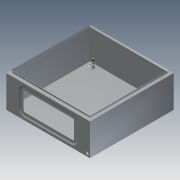
# Autodesk Inventor part: AE 1050_01_00
Saved by Autodesk Inventor 2016 (Build 200138000, 138)
## iProperties
Category: PARTsolutions
Company: RITTAL
Created: 2014-04-04
Part Number: AE 1050_01_00
Catalog Web Link: www.cadenas.de
Description: Gehäusekorpus AE-Gehäusekorpus AE
Vendor: RITTAL
Document SubType Name: Modeling
Designer: PARTuser1
Manufacturer: RITTAL
Density: 1 g/cm^3
Material: Generic
Appearance: RGB(195.00000357627781,201.00000321865156,196.00000351667384)
PSOL_IDENT_0: {$CADENAS_DATA\23d-libs\rittal\schaltschranksys\kompakt_schaltschr\ae\parts_ae\gehaeusekorpus_ae.prj
PSOL_IDENT_1: },187 {VTYP=3D},{NB=1050_01_00 (1)},{LINA=1050_01_00 (1)},{NN=Gehäusekorpus AE},{DATE=28.03.2014 09:
PSOL_IDENT_2: 17:10},{GEOMDATE=28.03.2014 09:16:00},{VERSION=},{LINEID=180},{LINESUBID=-1},{WBVAR=DETAIL}  {NB=105
PSOL_IDENT_3: 0_01_00 (1)},{LINA=1050_01_00 (1)},{KT=DUMMY},{BEST=1050},{VER=0},{SS=1.20},{DETAIL=1},{A=500.000},{
PSOL_IDENT_4: B=500.000},{C=210.000},{D=303.000},{E=113.000},{F=38.000},{G=30.000},{H=445.000},{I=355.000},{K=470.
PSOL_IDENT_5: 000},{P=410.000},{Q=449.000},{R=495.000},{S=495.000},{T=356.300},{U=425.000},{V=17.000},{W=438.000},
PSOL_IDENT_6: {X=411.000},{Y=423.000},{B1=500},{H1=500},{T1=210},{F1=449},{G1=470},{S1=2.5},{GEW=16.8},{VERS=1},{G
PSOL_IDENT_7: G=10.000},{AA=17.000},{BB=7.000},{CC=10.000},{RR=31.000}
CNS_NN: Gehäusekorpus AE
CNS_NT: Gehäusekorpus AE
CNS_NB: 1050_01_00 (1)
CNS_NBSYN: $BEST._01_00 ($DETAIL.)
CNS_LINA: 1050_01_00 (1)
CNS_BEST: 1050
CNS_VER: 0
CNS_SS: 1.20
CNS_DETAIL: 1
CNS_A: 500.000
CNS_B: 500.000
CNS_C: 210.000
CNS_D: 303.000
CNS_E: 113.000
CNS_F: 38.000
CNS_G: 30.000
CNS_H: 445.000
CNS_I: 355.000
CNS_K: 470.000
CNS_P: 410.000
CNS_Q: 449.000
CNS_R: 495.000
CNS_S: 495.000
CNS_T: 356.300
CNS_U: 425.000
CNS_V: 17.000
CNS_W: 438.000
CNS_X: 411.000
CNS_Y: 423.000
CNS_B1: 500
CNS_H1: 500
CNS_T1: 210
CNS_F1: 449
CNS_G1: 470
CNS_S1: 2.5
CNS_GEW: 16.8
CNS_VERS: 1
CNS_GG: 10.000
CNS_AA: 17.000
CNS_BB: 7.000
CNS_CC: 10.000
CNS_RR: 31.000
SUPPLIER: RITTAL
ARTICLENO: 1050_01_00 (1)
BOMINFO: 1050_01_00 (1)
CREATOR: CADENAS GmbH
Title: 1050_01_00 (1)
Author: Cadenas PARTsolutions
Comments: Gehäusekorpus AE
Autodesk Inventor part; units mm, degrees
sketch "Sketch_10" plane through (0, 0, 0) normal (0, 1, 0) x (-1, 0, 0)
  line L0 (250, -105) -> (250, 85)
  line L1 (250, 85) -> (-250, 85)
  line L2 (-250, 85) -> (-250, -105)
  line L3 (-250, -105) -> (250, -105)
  constraints: 8 end point
extrude "Extrusion1" add sketch "Sketch_10" along normal blind 500
sketch "Skizze_4" plane through (0, 0, 0) normal (1, 0, 0) x (0, 0, -1)
  line L0 (-210, 17) -> (0, 17)
  line L1 (0, 17) -> (0, 483)
  line L2 (0, 483) -> (-210, 483)
  line L3 (-210, 483) -> (-210, 17)
  constraints: 8 end point
extrude "Extrusion2" cut sketch "Skizze_4" along normal mid plane 465
sketch "Sketch_9" plane through (0, 0, 0) normal (1, 0, 0) x (0, 1, 0)
  line L0 (1.2, 83.8) -> (1.2, -103.8)
  line L1 (1.2, -103.8) -> (498.8, -103.8)
  line L2 (498.8, -103.8) -> (498.8, 83.8)
  line L3 (498.8, 83.8) -> (1.2, 83.8)
  constraints: 8 end point
extrude "Extrusion3" cut sketch "Sketch_9" along normal mid plane 497.6
sketch "Skizze_6" plane through (0, 0, 0) normal (1, 0, 0) x (0, 0, -1)
  line L0 (-103.9031, 11.333) -> (-103.9031, 10.1328)
  line L1 (-103.9031, 10.1328) -> (-83.8, 10.1328)
  line L2 (-83.8, 10.1328) -> (-83.8, 18)
  arc A0 (-83.8, 18) -> (-85.8, 20) centre (-85.8, 18) ccw
  line L3 (-85.8, 20) -> (-91.349, 20)
  arc A1 (-91.349, 20) -> (-92.5263, 19.6168) centre (-91.349, 18) ccw
  line L4 (-92.5263, 19.6168) -> (-103.9031, 11.333)
  constraints: 10 end point, 4 point on circle, 2 centre point
extrude "Extrusion4" add sketch "Skizze_6" along normal mid plane 478.4
sketch "Skizze_7" plane through (0, 0, 0) normal (1, 0, 0) x (0, 0, -1)
  line L0 (-103.9031, 488.667) -> (-92.5263, 480.3832)
  arc A0 (-92.5263, 480.3832) -> (-91.349, 480) centre (-91.349, 482) ccw
  line L1 (-91.349, 480) -> (-85.8, 480)
  arc A1 (-85.8, 480) -> (-83.8, 482) centre (-85.8, 482) ccw
  line L2 (-83.8, 482) -> (-83.8, 489.8672)
  line L3 (-83.8, 489.8672) -> (-103.9031, 489.8672)
  line L4 (-103.9031, 489.8672) -> (-103.9031, 488.667)
  constraints: 10 end point, 4 point on circle, 2 centre point
extrude "Extrusion5" add sketch "Skizze_7" along normal mid plane 476.4
sketch "Skizze_8" plane through (0, 250, 0) normal (0, 1, 0) x (1, 0, 0)
  line L0 (230, -85.8) -> (230, -91.349)
  arc A0 (230, -91.349) -> (230.3832, -92.5263) centre (232, -91.349) ccw
  line L1 (230.3832, -92.5263) -> (238.667, -103.9031)
  line L2 (238.667, -103.9031) -> (239.867, -103.9031)
  line L3 (239.867, -103.9031) -> (239.867, -83.8)
  line L4 (239.867, -83.8) -> (232, -83.8)
  arc A1 (232, -83.8) -> (230, -85.8) centre (232, -85.8) ccw
  constraints: 10 end point, 4 point on circle, 2 centre point
extrude "Extrusion6" add sketch "Skizze_8" along normal mid plane 481.4
sketch "Skizze_9" plane through (0, 250, 0) normal (0, 1, 0) x (1, 0, 0)
  line L0 (-240.6254, -103.9031) -> (-238.667, -103.9031)
  line L1 (-238.667, -103.9031) -> (-230.3832, -92.5263)
  arc A0 (-230.3832, -92.5263) -> (-230, -91.349) centre (-232, -91.349) ccw
  line L2 (-230, -91.349) -> (-230, -85.8)
  arc A1 (-230, -85.8) -> (-232, -83.8) centre (-232, -85.8) ccw
  line L3 (-232, -83.8) -> (-240.6254, -83.8)
  line L4 (-240.6254, -83.8) -> (-240.6254, -103.9031)
  constraints: 10 end point, 4 point on circle, 2 centre point
extrude "Extrusion7" add sketch "Skizze_9" along normal mid plane 481.4
sketch "Skizze_20" plane through (0, 0, 0) normal (1, 0, 0) x (0, 0, -1)
  line L0 (-296.7396, -2) -> (-85, -2)
  line L1 (-85, -2) -> (-85, 18)
  arc A0 (-85, 18) -> (-85.8, 18.8) centre (-85.8, 18) ccw
  line L2 (-85.8, 18.8) -> (-91.3601, 18.8)
  arc A1 (-91.3601, 18.8) -> (-91.8245, 18.6514) centre (-91.3601, 18) ccw
  line L3 (-91.8245, 18.6514) -> (-98.7083, 13.7444)
  line L4 (-98.7083, 13.7444) -> (-276.7396, 250)
  line L5 (-276.7396, 250) -> (-98.7083, 486.2556)
  line L6 (-98.7083, 486.2556) -> (-91.8245, 481.3486)
  arc A2 (-91.8245, 481.3486) -> (-91.3601, 481.2) centre (-91.3601, 482) ccw
  line L7 (-91.3601, 481.2) -> (-85.8, 481.2)
  arc A3 (-85.8, 481.2) -> (-85, 482) centre (-85.8, 482) ccw
  line L8 (-85, 482) -> (-85, 502)
  line L9 (-85, 502) -> (-296.7396, 502)
  line L10 (-296.7396, 502) -> (-296.7396, -2)
  constraints: 22 end point, 8 point on circle, 4 centre point
extrude "Extrusion8" cut sketch "Skizze_20" along normal mid plane 1476.4
sketch "Skizze_21" plane through (0, 250, 0) normal (0, 1, 0) x (1, 0, 0)
  line L0 (-251.2, -85) -> (-251.2, -296.7396)
  line L1 (-251.2, -296.7396) -> (251.2, -296.7396)
  line L2 (251.2, -296.7396) -> (251.2, -85)
  line L3 (251.2, -85) -> (232, -85)
  arc A0 (232, -85) -> (231.2, -85.8) centre (232, -85.8) ccw
  line L4 (231.2, -85.8) -> (231.2, -91.3601)
  arc A1 (231.2, -91.3601) -> (231.3486, -91.8245) centre (232, -91.3601) ccw
  line L5 (231.3486, -91.8245) -> (236.2556, -98.7083)
  line L6 (236.2556, -98.7083) -> (0, -276.7396)
  line L7 (0, -276.7396) -> (-236.2556, -98.7083)
  line L8 (-236.2556, -98.7083) -> (-231.3486, -91.8245)
  arc A2 (-231.3486, -91.8245) -> (-231.2, -91.3601) centre (-232, -91.3601) ccw
  line L9 (-231.2, -91.3601) -> (-231.2, -85.8)
  arc A3 (-231.2, -85.8) -> (-232, -85) centre (-232, -85.8) ccw
  line L10 (-232, -85) -> (-251.2, -85)
  constraints: 22 end point, 8 point on circle, 4 centre point
extrude "Extrusion9" cut sketch "Skizze_21" along normal mid plane 496.4
sketch "Sketch10" plane through (-250, 0, 85) normal (0, 0, 1) x (1, 0, 0)
  point P0 (490.3, 50.65)
hole "Drilling 1" at (240.3, 50.65, 85) direction (0, 0, -1) diameter 4.4 depth 1.2
sketch "Skizze_28" plane through (0, 0, 0) normal (0, 1, 0) x (1, 0, 0)
  line L0 (-182.9449, 50.4449) -> (-182.9449, -29.4449)
  arc A0 (-182.9449, -29.4449) -> (-134.9449, -77.4449) centre (-134.9449, -29.4449) ccw
  line L1 (-134.9449, -77.4449) -> (134.9449, -77.4449)
  arc A1 (134.9449, -77.4449) -> (182.9449, -29.4449) centre (134.9449, -29.4449) ccw
  line L2 (182.9449, -29.4449) -> (182.9449, 50.4449)
  arc A2 (182.9449, 50.4449) -> (134.9449, 98.4449) centre (134.9449, 50.4449) ccw
  line L3 (134.9449, 98.4449) -> (-134.9449, 98.4449)
  arc A3 (-134.9449, 98.4449) -> (-182.9449, 50.4449) centre (-134.9449, 50.4449) ccw
  constraints: 8 end point, 8 point on circle, 4 centre point
extrude "Extrusion10" cut sketch "Skizze_28" along normal blind 1.2
sketch "Skizze_29" plane through (0, 0, -10.5) normal (0, 0, 1) x (1, 0, 0)
  line L0 (147.5, 4) -> (167.6962, 4)
  arc A0 (168.5962, 3.7588) -> (167.6962, 4) centre (167.6962, 2.2) ccw
  line L1 (168.5962, 3.7588) -> (174.4105, 0.4019)
  arc A1 (174.4105, 0.4019) -> (175.9105, 0) centre (175.9105, 3) ccw
  line L2 (175.9105, 0) -> (182.9949, 0)
  line L3 (182.9949, 0) -> (182.9949, 1.2)
  line L4 (182.9949, 1.2) -> (175.9105, 1.2)
  arc A2 (175.0105, 1.4412) -> (175.9105, 1.2) centre (175.9105, 3) ccw
  line L5 (175.0105, 1.4412) -> (169.1962, 4.7981)
  arc A3 (169.1962, 4.7981) -> (167.6962, 5.2) centre (167.6962, 2.2) ccw
  line L6 (167.6962, 5.2) -> (147.5, 5.2)
  line L7 (147.5, 5.2) -> (147.5, 4)
  constraints: 16 end point, 8 point on circle, 4 centre point
extrude "Extrusion11" add sketch "Skizze_29" along normal mid plane 85
sketch "Skizze_30" plane through (0, 0, -10.5) normal (0, 0, 1) x (1, 0, 0)
  line L0 (-182.9949, 0) -> (-175.9105, 0)
  arc A0 (-175.9105, 0) -> (-174.4105, 0.4019) centre (-175.9105, 3) ccw
  line L1 (-174.4105, 0.4019) -> (-168.5962, 3.7588)
  arc A1 (-167.6962, 4) -> (-168.5962, 3.7588) centre (-167.6962, 2.2) ccw
  line L2 (-167.6962, 4) -> (-147.5, 4)
  line L3 (-147.5, 4) -> (-147.5, 5.2)
  line L4 (-147.5, 5.2) -> (-167.6962, 5.2)
  arc A2 (-167.6962, 5.2) -> (-169.1962, 4.7981) centre (-167.6962, 2.2) ccw
  line L5 (-169.1962, 4.7981) -> (-175.0105, 1.4412)
  arc A3 (-175.9105, 1.2) -> (-175.0105, 1.4412) centre (-175.9105, 3) ccw
  line L6 (-175.9105, 1.2) -> (-182.9949, 1.2)
  line L7 (-182.9949, 1.2) -> (-182.9949, 0)
  constraints: 16 end point, 8 point on circle, 4 centre point
extrude "Extrusion12" add sketch "Skizze_30" along normal mid plane 85
sketch "Skizze_31" plane through (0, 0, -53) normal (0, 0, 1) x (1, 0, 0)
  line L0 (137.5, -50) -> (137.5, 50)
  line L1 (147.5, 4) -> (167.6962, 4)
  arc A0 (168.5962, 3.7588) -> (167.6962, 4) centre (167.6962, 2.2) ccw
  line L2 (168.5962, 3.7588) -> (174.4105, 0.4019)
  arc A1 (174.4105, 0.4019) -> (175.9105, 0) centre (175.9105, 3) ccw
  line L3 (175.9105, 0) -> (182.9949, 0)
  line L4 (182.9949, 0) -> (182.9949, 1.2)
  line L5 (182.9949, 1.2) -> (175.9105, 1.2)
  arc A2 (175.0105, 1.4412) -> (175.9105, 1.2) centre (175.9105, 3) ccw
  line L6 (175.0105, 1.4412) -> (169.1962, 4.7981)
  arc A3 (169.1962, 4.7981) -> (167.6962, 5.2) centre (167.6962, 2.2) ccw
  line L7 (167.6962, 5.2) -> (147.5, 5.2)
  line L8 (147.5, 5.2) -> (147.5, 4)
  constraints: 18 end point, 8 point on circle, 4 centre point
revolve "Revolution1" add sketch "Skizze_31" angle 90 about axis through (137.5, -50, -53) along (0, 1, 0)
sketch "Skizze_32" plane through (0, 0, -53) normal (0, 0, 1) x (1, 0, 0)
  line L0 (-137.5, 4) -> (-137.5, -4)
  line L1 (-182.9949, 0) -> (-175.9105, 0)
  arc A0 (-175.9105, 0) -> (-174.4105, 0.4019) centre (-175.9105, 3) ccw
  line L2 (-174.4105, 0.4019) -> (-168.5962, 3.7588)
  arc A1 (-167.6962, 4) -> (-168.5962, 3.7588) centre (-167.6962, 2.2) ccw
  line L3 (-167.6962, 4) -> (-147.5, 4)
  line L4 (-147.5, 4) -> (-147.5, 5.2)
  line L5 (-147.5, 5.2) -> (-167.6962, 5.2)
  arc A2 (-167.6962, 5.2) -> (-169.1962, 4.7981) centre (-167.6962, 2.2) ccw
  line L6 (-169.1962, 4.7981) -> (-175.0105, 1.4412)
  arc A3 (-175.9105, 1.2) -> (-175.0105, 1.4412) centre (-175.9105, 3) ccw
  line L7 (-175.9105, 1.2) -> (-182.9949, 1.2)
  line L8 (-182.9949, 1.2) -> (-182.9949, 0)
  constraints: 18 end point, 8 point on circle, 4 centre point
revolve "Revolution2" add sketch "Skizze_32" angle 90 about axis through (-137.5, 4, -53) along (0, -1, 0)
sketch "Skizze_33" plane through (0, 0, 32) normal (0, 0, 1) x (1, 0, 0)
  line L0 (137.5, -50) -> (137.5, 50)
  line L1 (147.5, 4) -> (167.6962, 4)
  arc A0 (168.5962, 3.7588) -> (167.6962, 4) centre (167.6962, 2.2) ccw
  line L2 (168.5962, 3.7588) -> (174.4105, 0.4019)
  arc A1 (174.4105, 0.4019) -> (175.9105, 0) centre (175.9105, 3) ccw
  line L3 (175.9105, 0) -> (182.9949, 0)
  line L4 (182.9949, 0) -> (182.9949, 1.2)
  line L5 (182.9949, 1.2) -> (175.9105, 1.2)
  arc A2 (175.0105, 1.4412) -> (175.9105, 1.2) centre (175.9105, 3) ccw
  line L6 (175.0105, 1.4412) -> (169.1962, 4.7981)
  arc A3 (169.1962, 4.7981) -> (167.6962, 5.2) centre (167.6962, 2.2) ccw
  line L7 (167.6962, 5.2) -> (147.5, 5.2)
  line L8 (147.5, 5.2) -> (147.5, 4)
  constraints: 18 end point, 8 point on circle, 4 centre point
revolve "Revolution3" add sketch "Skizze_33" angle 90 about axis through (137.5, -50, 32) along (0, -1, 0)
sketch "Skizze_34" plane through (0, 0, 32) normal (0, 0, 1) x (1, 0, 0)
  line L0 (-137.5, 4) -> (-137.5, -4)
  line L1 (-182.9949, 0) -> (-175.9105, 0)
  arc A0 (-175.9105, 0) -> (-174.4105, 0.4019) centre (-175.9105, 3) ccw
  line L2 (-174.4105, 0.4019) -> (-168.5962, 3.7588)
  arc A1 (-167.6962, 4) -> (-168.5962, 3.7588) centre (-167.6962, 2.2) ccw
  line L3 (-167.6962, 4) -> (-147.5, 4)
  line L4 (-147.5, 4) -> (-147.5, 5.2)
  line L5 (-147.5, 5.2) -> (-167.6962, 5.2)
  arc A2 (-167.6962, 5.2) -> (-169.1962, 4.7981) centre (-167.6962, 2.2) ccw
  line L6 (-169.1962, 4.7981) -> (-175.0105, 1.4412)
  arc A3 (-175.9105, 1.2) -> (-175.0105, 1.4412) centre (-175.9105, 3) ccw
  line L7 (-175.9105, 1.2) -> (-182.9949, 1.2)
  line L8 (-182.9949, 1.2) -> (-182.9949, 0)
  constraints: 18 end point, 8 point on circle, 4 centre point
revolve "Revolution4" add sketch "Skizze_34" angle 90 about axis through (-137.5, 4, 32) along (0, 1, 0)
sketch "Skizze_35" plane through (0, 0, 0) normal (1, 0, 0) x (0, 0, -1)
  line L0 (63, 4) -> (83.1962, 4)
  arc A0 (84.0962, 3.7588) -> (83.1962, 4) centre (83.1962, 2.2) ccw
  line L1 (84.0962, 3.7588) -> (89.9105, 0.4019)
  arc A1 (89.9105, 0.4019) -> (91.4105, 0) centre (91.4105, 3) ccw
  line L2 (91.4105, 0) -> (98.4949, 0)
  line L3 (98.4949, 0) -> (98.4949, 1.2)
  line L4 (98.4949, 1.2) -> (91.4105, 1.2)
  arc A2 (90.5105, 1.4412) -> (91.4105, 1.2) centre (91.4105, 3) ccw
  line L5 (90.5105, 1.4412) -> (84.6962, 4.7981)
  arc A3 (84.6962, 4.7981) -> (83.1962, 5.2) centre (83.1962, 2.2) ccw
  line L6 (83.1962, 5.2) -> (63, 5.2)
  line L7 (63, 5.2) -> (63, 4)
  constraints: 16 end point, 8 point on circle, 4 centre point
extrude "Extrusion13" add sketch "Skizze_35" along normal mid plane 275
sketch "Skizze_36" plane through (0, 0, 0) normal (1, 0, 0) x (0, 0, -1)
  line L0 (-77.4949, 0) -> (-70.4105, 0)
  arc A0 (-70.4105, 0) -> (-68.9105, 0.4019) centre (-70.4105, 3) ccw
  line L1 (-68.9105, 0.4019) -> (-63.0962, 3.7588)
  arc A1 (-62.1962, 4) -> (-63.0962, 3.7588) centre (-62.1962, 2.2) ccw
  line L2 (-62.1962, 4) -> (-42, 4)
  line L3 (-42, 4) -> (-42, 5.2)
  line L4 (-42, 5.2) -> (-62.1962, 5.2)
  arc A2 (-62.1962, 5.2) -> (-63.6962, 4.7981) centre (-62.1962, 2.2) ccw
  line L5 (-63.6962, 4.7981) -> (-69.5105, 1.4412)
  arc A3 (-70.4105, 1.2) -> (-69.5105, 1.4412) centre (-70.4105, 3) ccw
  line L6 (-70.4105, 1.2) -> (-77.4949, 1.2)
  line L7 (-77.4949, 1.2) -> (-77.4949, 0)
  constraints: 16 end point, 8 point on circle, 4 centre point
extrude "Extrusion14" add sketch "Skizze_36" along normal mid plane 275
sketch "Skizze_105" plane through (0, 5.2, 0) normal (0, 1, 0) x (1, 0, 0)
  line L0 (-151.5, 67) -> (-151.5, -46)
  line L1 (-151.5, -46) -> (151.5, -46)
  line L2 (151.5, -46) -> (151.5, 67)
  line L3 (151.5, 67) -> (-151.5, 67)
  constraints: 8 end point
extrude "Extrusion15" add sketch "Skizze_105" against normal blind 1.2
sketch "Skizze_106" plane through (0, 5.2, 0) normal (0, 1, 0) x (1, 0, 0)
  line L0 (-151.5, 59) -> (-151.5, -38)
  arc A0 (-151.5, -38) -> (-143.5, -46) centre (-143.5, -38) ccw
  line L1 (-143.5, -46) -> (143.5, -46)
  arc A1 (143.5, -46) -> (151.5, -38) centre (143.5, -38) ccw
  line L2 (151.5, -38) -> (151.5, 59)
  arc A2 (151.5, 59) -> (143.5, 67) centre (143.5, 59) ccw
  line L3 (143.5, 67) -> (-143.5, 67)
  arc A3 (-143.5, 67) -> (-151.5, 59) centre (-143.5, 59) ccw
  constraints: 8 end point, 8 point on circle, 4 centre point
extrude "Extrusion16" cut sketch "Skizze_106" against normal blind 1.2
sketch "Skizze_48" plane through (0, 0, -103.8) normal (0, 0, 1) x (1, 0, 0)
  line L0 (196, 39.3808) -> (196, 20.6192)
  arc A0 (196, 20.6192) -> (214, 20.6192) centre (205, 30) ccw
  line L1 (214, 20.6192) -> (214, 39.3808)
  arc A1 (214, 39.3808) -> (196, 39.3808) centre (205, 30) ccw
  circle A2 centre (210, 38) radius 2
  circle A3 centre (210, 22) radius 2
  circle A4 centre (200, 38) radius 2
  circle A5 centre (200, 22) radius 2
  constraints: 6 centre point, 4 end point, 4 point on circle
extrude "Extrusion17" add sketch "Skizze_48" along normal blind 1.8
sketch "Skizze_49" plane through (0, 0, -103.8) normal (0, 0, 1) x (1, 0, 0)
  line L0 (-214, 39.3808) -> (-214, 20.6192)
  arc A0 (-214, 20.6192) -> (-196, 20.6192) centre (-205, 30) ccw
  line L1 (-196, 20.6192) -> (-196, 39.3808)
  arc A1 (-196, 39.3808) -> (-214, 39.3808) centre (-205, 30) ccw
  circle A2 centre (-200, 38) radius 2
  circle A3 centre (-200, 22) radius 2
  circle A4 centre (-210, 38) radius 2
  circle A5 centre (-210, 22) radius 2
  constraints: 6 centre point, 4 end point, 4 point on circle
extrude "Extrusion18" add sketch "Skizze_49" along normal blind 1.8
sketch "Skizze_50" plane through (0, 0, -103.8) normal (0, 0, 1) x (1, 0, 0)
  line L0 (196, 484.3808) -> (196, 465.6192)
  arc A0 (196, 465.6192) -> (214, 465.6192) centre (205, 475) ccw
  line L1 (214, 465.6192) -> (214, 484.3808)
  arc A1 (214, 484.3808) -> (196, 484.3808) centre (205, 475) ccw
  circle A2 centre (210, 483) radius 2
  circle A3 centre (210, 467) radius 2
  circle A4 centre (200, 483) radius 2
  circle A5 centre (200, 467) radius 2
  constraints: 6 centre point, 4 end point, 4 point on circle
extrude "Extrusion19" add sketch "Skizze_50" along normal blind 1.8
sketch "Skizze_51" plane through (0, 0, -103.8) normal (0, 0, 1) x (1, 0, 0)
  line L0 (-214, 484.3808) -> (-214, 465.6192)
  arc A0 (-214, 465.6192) -> (-196, 465.6192) centre (-205, 475) ccw
  line L1 (-196, 465.6192) -> (-196, 484.3808)
  arc A1 (-196, 484.3808) -> (-214, 484.3808) centre (-205, 475) ccw
  circle A2 centre (-200, 483) radius 2
  circle A3 centre (-200, 467) radius 2
  circle A4 centre (-210, 483) radius 2
  circle A5 centre (-210, 467) radius 2
  constraints: 6 centre point, 4 end point, 4 point on circle
extrude "Extrusion20" add sketch "Skizze_51" along normal blind 1.8
sketch "Skizze_47" plane through (205, 0, 0) normal (1, 0, 0) x (0, 0, -1)
  line L0 (102, 30) -> (55, 30)
  line L1 (55, 30) -> (55, 33.233)
  line L2 (55, 33.233) -> (55.767, 34)
  line L3 (55.767, 34) -> (77.9347, 34)
  line L4 (77.9347, 34) -> (79.8, 39.125)
  line L5 (79.8, 39.125) -> (81, 39.125)
  line L6 (81, 39.125) -> (81, 34)
  line L7 (81, 34) -> (86, 34)
  line L8 (86, 34) -> (86, 38.65)
  line L9 (86, 38.65) -> (88, 38.65)
  line L10 (88, 38.65) -> (88, 35.325)
  line L11 (88, 35.325) -> (93.6, 35.325)
  line L12 (93.6, 35.325) -> (93.6, 35.1)
  line L13 (93.6, 35.1) -> (102, 35.1)
  line L14 (102, 35.1) -> (102, 30)
  line L15 (102, 30) -> (55, 30)
  constraints: 32 end point
revolve "Revolution5" add sketch "Skizze_47" angle 360 about axis through (205, 30, -102) along (0, 0, -1)
thread "Thread1" size "M8x1.25" class "6g" standard "ISO Metric profile" full length
sketch "Skizze_53" plane through (205, 0, 0) normal (1, 0, 0) x (0, 0, -1)
  line L0 (102, 475) -> (55, 475)
  line L1 (55, 475) -> (55, 478.233)
  line L2 (55, 478.233) -> (55.767, 479)
  line L3 (55.767, 479) -> (77.9347, 479)
  line L4 (77.9347, 479) -> (79.8, 484.125)
  line L5 (79.8, 484.125) -> (81, 484.125)
  line L6 (81, 484.125) -> (81, 479)
  line L7 (81, 479) -> (86, 479)
  line L8 (86, 479) -> (86, 483.65)
  line L9 (86, 483.65) -> (88, 483.65)
  line L10 (88, 483.65) -> (88, 480.325)
  line L11 (88, 480.325) -> (93.6, 480.325)
  line L12 (93.6, 480.325) -> (93.6, 480.1)
  line L13 (93.6, 480.1) -> (102, 480.1)
  line L14 (102, 480.1) -> (102, 475)
  line L15 (102, 475) -> (55, 475)
  constraints: 32 end point
revolve "Revolution6" add sketch "Skizze_53" angle 360 about axis through (205, 475, -102) along (0, 0, -1)
thread "Thread2" size "M8x1.25" class "6g" standard "ISO Metric profile" full length
sketch "Skizze_55" plane through (-205, 0, 0) normal (1, 0, 0) x (0, 0, -1)
  line L0 (102, 30) -> (55, 30)
  line L1 (55, 30) -> (55, 33.233)
  line L2 (55, 33.233) -> (55.767, 34)
  line L3 (55.767, 34) -> (77.9347, 34)
  line L4 (77.9347, 34) -> (79.8, 39.125)
  line L5 (79.8, 39.125) -> (81, 39.125)
  line L6 (81, 39.125) -> (81, 34)
  line L7 (81, 34) -> (86, 34)
  line L8 (86, 34) -> (86, 38.65)
  line L9 (86, 38.65) -> (88, 38.65)
  line L10 (88, 38.65) -> (88, 35.325)
  line L11 (88, 35.325) -> (93.6, 35.325)
  line L12 (93.6, 35.325) -> (93.6, 35.1)
  line L13 (93.6, 35.1) -> (102, 35.1)
  line L14 (102, 35.1) -> (102, 30)
  line L15 (102, 30) -> (55, 30)
  constraints: 32 end point
revolve "Revolution7" add sketch "Skizze_55" angle 360 about axis through (-205, 30, -102) along (0, 0, -1)
thread "Thread3" size "M8x1.25" class "6g" standard "ISO Metric profile" full length
sketch "Skizze_57" plane through (-205, 0, 0) normal (1, 0, 0) x (0, 0, -1)
  line L0 (102, 475) -> (55, 475)
  line L1 (55, 475) -> (55, 478.233)
  line L2 (55, 478.233) -> (55.767, 479)
  line L3 (55.767, 479) -> (77.9347, 479)
  line L4 (77.9347, 479) -> (79.8, 484.125)
  line L5 (79.8, 484.125) -> (81, 484.125)
  line L6 (81, 484.125) -> (81, 479)
  line L7 (81, 479) -> (86, 479)
  line L8 (86, 479) -> (86, 483.65)
  line L9 (86, 483.65) -> (88, 483.65)
  line L10 (88, 483.65) -> (88, 480.325)
  line L11 (88, 480.325) -> (93.6, 480.325)
  line L12 (93.6, 480.325) -> (93.6, 480.1)
  line L13 (93.6, 480.1) -> (102, 480.1)
  line L14 (102, 480.1) -> (102, 475)
  line L15 (102, 475) -> (55, 475)
  constraints: 32 end point
revolve "Revolution8" add sketch "Skizze_57" angle 360 about axis through (-205, 475, -102) along (0, 0, -1)
thread "Thread4" size "M8x1.25" class "6g" standard "ISO Metric profile" full length
sketch "Sketch30" plane through (0, 0, 0) normal (0, -1, 0) x (1, 0, 0)
  point P0 (233.5, -88.5)
hole "Drilling 2" at (233.5, 0, -88.5) direction (0, 1, 0) diameter 16 depth 1.2
sketch "Sketch31" plane through (250, 0, -105) normal (0, 0, -1) x (-1, 0, 0)
  point P0 (20, 20)
hole "Drilling 3" at (230, 20, -105) direction (0, 0, 1) diameter 24 depth 1.2
sketch "Sketch32" plane through (250, 0, -105) normal (0, 0, -1) x (-1, 0, 0)
  point P0 (20, 480)
hole "Drilling 4" at (230, 480, -105) direction (0, 0, 1) diameter 24 depth 1.2
sketch "Skizze_69" plane through (230, 0, 0) normal (1, 0, 0) x (0, 0, -1)
  line L0 (105, 20) -> (101.8, 20)
  line L1 (101.8, 20) -> (101.8, 27.3373)
  arc A0 (102.6201, 29.3172) -> (101.8, 27.3373) centre (104.6, 27.3373) ccw
  line L2 (102.6201, 29.3172) -> (103.3314, 30.0284)
  arc A1 (103.3314, 30.0284) -> (103.8, 31.1598) centre (102.2, 31.1598) ccw
  line L3 (103.8, 31.1598) -> (103.8, 32.5)
  line L4 (103.8, 32.5) -> (105, 32.5)
  line L5 (105, 32.5) -> (105, 31.1598)
  arc A2 (104.1799, 29.1799) -> (105, 31.1598) centre (102.2, 31.1598) ccw
  line L6 (104.1799, 29.1799) -> (103.4686, 28.4686)
  arc A3 (103.4686, 28.4686) -> (103, 27.3373) centre (104.6, 27.3373) ccw
  line L7 (103, 27.3373) -> (103, 20)
  line L8 (103, 20) -> (101.8, 20)
  constraints: 18 end point, 8 point on circle, 4 centre point
revolve "Revolution9" add sketch "Skizze_69" angle 360 about axis through (230, 20, -105) along (0, 0, -1)
sketch "Skizze_72" plane through (230, 0, 0) normal (1, 0, 0) x (0, 0, -1)
  line L0 (105, 480) -> (103.8, 480)
  line L1 (101.8, 480) -> (101.8, 487.3373)
  arc A0 (102.6201, 489.3172) -> (101.8, 487.3373) centre (104.6, 487.3373) ccw
  line L2 (102.6201, 489.3172) -> (103.3314, 490.0284)
  arc A1 (103.3314, 490.0284) -> (103.8, 491.1598) centre (102.2, 491.1598) ccw
  line L3 (103.8, 491.1598) -> (103.8, 492.5)
  line L4 (103.8, 492.5) -> (105, 492.5)
  line L5 (105, 492.5) -> (105, 491.1598)
  arc A2 (104.1799, 489.1799) -> (105, 491.1598) centre (102.2, 491.1598) ccw
  line L6 (104.1799, 489.1799) -> (103.4686, 488.4686)
  arc A3 (103.4686, 488.4686) -> (103, 487.3373) centre (104.6, 487.3373) ccw
  line L7 (103, 487.3373) -> (103, 480)
  line L8 (103, 480) -> (101.8, 480)
  constraints: 18 end point, 8 point on circle, 4 centre point
revolve "Revolution10" add sketch "Skizze_72" angle 360 about axis through (230, 480, -105) along (0, 0, -1)
sketch "Sketch35" plane through (250, 0, -105) normal (0, 0, -1) x (-1, 0, 0)
  point P0 (480, 20)
hole "Drilling 5" at (-230, 20, -105) direction (0, 0, 1) diameter 24 depth 1.2
sketch "Sketch36" plane through (250, 0, -105) normal (0, 0, -1) x (-1, 0, 0)
  point P0 (480, 480)
hole "Drilling 6" at (-230, 480, -105) direction (0, 0, 1) diameter 24 depth 1.2
sketch "Skizze_77" plane through (-230, 0, 0) normal (1, 0, 0) x (0, 0, -1)
  line L0 (105, 20) -> (103.8, 20)
  line L1 (101.8, 20) -> (101.8, 27.3373)
  arc A0 (102.6201, 29.3172) -> (101.8, 27.3373) centre (104.6, 27.3373) ccw
  line L2 (102.6201, 29.3172) -> (103.3314, 30.0284)
  arc A1 (103.3314, 30.0284) -> (103.8, 31.1598) centre (102.2, 31.1598) ccw
  line L3 (103.8, 31.1598) -> (103.8, 32.5)
  line L4 (103.8, 32.5) -> (105, 32.5)
  line L5 (105, 32.5) -> (105, 31.1598)
  arc A2 (104.1799, 29.1799) -> (105, 31.1598) centre (102.2, 31.1598) ccw
  line L6 (104.1799, 29.1799) -> (103.4686, 28.4686)
  arc A3 (103.4686, 28.4686) -> (103, 27.3373) centre (104.6, 27.3373) ccw
  line L7 (103, 27.3373) -> (103, 20)
  line L8 (103, 20) -> (101.8, 20)
  constraints: 18 end point, 8 point on circle, 4 centre point
revolve "Revolution11" add sketch "Skizze_77" angle 360 about axis through (-230, 20, -105) along (0, 0, -1)
sketch "Skizze_78" plane through (-230, 0, 0) normal (1, 0, 0) x (0, 0, -1)
  line L0 (105, 480) -> (103.8, 480)
  line L1 (101.8, 480) -> (101.8, 487.3373)
  arc A0 (102.6201, 489.3172) -> (101.8, 487.3373) centre (104.6, 487.3373) ccw
  line L2 (102.6201, 489.3172) -> (103.3314, 490.0284)
  arc A1 (103.3314, 490.0284) -> (103.8, 491.1598) centre (102.2, 491.1598) ccw
  line L3 (103.8, 491.1598) -> (103.8, 492.5)
  line L4 (103.8, 492.5) -> (105, 492.5)
  line L5 (105, 492.5) -> (105, 491.1598)
  arc A2 (104.1799, 489.1799) -> (105, 491.1598) centre (102.2, 491.1598) ccw
  line L6 (104.1799, 489.1799) -> (103.4686, 488.4686)
  arc A3 (103.4686, 488.4686) -> (103, 487.3373) centre (104.6, 487.3373) ccw
  line L7 (103, 487.3373) -> (103, 480)
  line L8 (103, 480) -> (101.8, 480)
  constraints: 18 end point, 8 point on circle, 4 centre point
revolve "Revolution12" add sketch "Skizze_78" angle 360 about axis through (-230, 480, -105) along (0, 0, -1)
sketch "Sketch_3" plane through (-230, 0, 0) normal (1, 0, 0) x (0, 0, -1)
  line L0 (105, 20) -> (101.8, 20)
  line L1 (101.8, 20) -> (101.8, 24.35)
  line L2 (101.8, 24.35) -> (105, 24.35)
  line L3 (105, 24.35) -> (105, 20)
  line L4 (105, 20) -> (101.8, 20)
  constraints: 10 end point
revolve "Revolution13" cut sketch "Sketch_3" angle 360 about axis through (-230, 20, -105) along (0, 0, -1)
sketch "Sketch_4" plane through (230, 0, 0) normal (1, 0, 0) x (0, 0, -1)
  line L0 (105, 20) -> (101.8, 20)
  line L1 (101.8, 20) -> (101.8, 24.35)
  line L2 (101.8, 24.35) -> (105, 24.35)
  line L3 (105, 24.35) -> (105, 20)
  line L4 (105, 20) -> (101.8, 20)
  constraints: 10 end point
revolve "Revolution14" cut sketch "Sketch_4" angle 360 about axis through (230, 20, -105) along (0, 0, -1)
sketch "Sketch_5" plane through (230, 0, 0) normal (1, 0, 0) x (0, 0, -1)
  line L0 (105, 480) -> (101.8, 480)
  line L1 (101.8, 480) -> (101.8, 484.35)
  line L2 (101.8, 484.35) -> (105, 484.35)
  line L3 (105, 484.35) -> (105, 480)
  line L4 (105, 480) -> (101.8, 480)
  constraints: 10 end point
revolve "Revolution15" cut sketch "Sketch_5" angle 360 about axis through (230, 480, -105) along (0, 0, -1)
sketch "Sketch_2" plane through (-230, 0, 0) normal (1, 0, 0) x (0, 0, -1)
  line L0 (105, 480) -> (101.8, 480)
  line L1 (101.8, 480) -> (101.8, 484.35)
  line L2 (101.8, 484.35) -> (105, 484.35)
  line L3 (105, 484.35) -> (105, 480)
  line L4 (105, 480) -> (101.8, 480)
  constraints: 10 end point
revolve "Revolution16" cut sketch "Sketch_2" angle 360 about axis through (-230, 480, -105) along (0, 0, -1)
sketch "Skizze_54" plane through (0, 0, 15) normal (0, 0, 1) x (1, 0, 0)
  line L0 (248.8, 30) -> (230.6, 30)
  line L1 (230.6, 30) -> (230.6, 33.233)
  line L2 (230.6, 33.233) -> (231.367, 34)
  line L3 (231.367, 34) -> (245.6, 34)
  line L4 (245.6, 34) -> (245.6, 40)
  line L5 (245.6, 40) -> (248.8, 40)
  line L6 (248.8, 40) -> (248.8, 30)
  line L7 (248.8, 30) -> (230.6, 30)
  constraints: 16 end point
revolve "Revolution17" add sketch "Skizze_54" angle 360 about axis through (248.8, 30, 15) along (1, 0, 0)
thread "Thread5" size "M8x1.25" class "6g" standard "ISO Metric profile" length 14 offset 1
sketch "Sketch44" plane through (167.6962, 5.2, 32) normal (0, 1, 0) x (1, 0, 0)
  point P0 (-287.6962, -24)
hole "Drilling 11" at (-120, 5.2, 56) direction (0, -1, 0) diameter 4 depth 1.2
pattern_linear "Rectangular Pattern1" count 3 spacing 120 along (1, 0, 0) of "Drilling 11"
sketch "Sketch45" plane through (167.6962, 5.2, 32) normal (0, 1, 0) x (1, 0, 0)
  point P0 (-287.6962, 109)
hole "Drilling 12" at (-120, 5.2, -77) direction (0, -1, 0) diameter 4 depth 1.2
pattern_linear "Rectangular Pattern2" count 3 spacing 120 along (1, 0, 0) of "Drilling 12"
sketch "Sketch46" plane through (167.6962, 5.2, 32) normal (0, 1, 0) x (1, 0, 0)
  point P0 (-329.1962, 42.5)
hole "Drilling 13" at (-161.5, 5.2, -10.5) direction (0, -1, 0) diameter 4 depth 1.2
sketch "Sketch47" plane through (167.6962, 5.2, 32) normal (0, 1, 0) x (1, 0, 0)
  point P0 (-6.1962, 42.5)
hole "Drilling 14" at (161.5, 5.2, -10.5) direction (0, -1, 0) diameter 4 depth 1.2
sketch "Sketch48" plane through (-250, 0, 85) normal (0, 0, 1) x (1, 0, 0)
  point P0 (490.3, 68.15)
hole "Drilling 15" at (240.3, 68.15, 85) direction (0, 0, -1) diameter 4.4 depth 1.2
sketch "Sketch49" plane through (-250, 0, 85) normal (0, 0, 1) x (1, 0, 0)
  point P0 (490.3, 431.85)
hole "Drilling 16" at (240.3, 431.85, 85) direction (0, 0, -1) diameter 4.4 depth 1.2
sketch "Sketch50" plane through (-250, 0, 85) normal (0, 0, 1) x (1, 0, 0)
  point P0 (490.3, 449.35)
hole "Drilling 17" at (240.3, 449.35, 85) direction (0, 0, -1) diameter 4.4 depth 1.2
sketch "Sketch_27" plane through (0, 0, -80) normal (0, 0, 1) x (1, 0, 0)
  line L0 (197.4944, 30) -> (201.2472, 23.5)
  line L1 (201.2472, 23.5) -> (208.7528, 23.5)
  line L2 (208.7528, 23.5) -> (212.5056, 30)
  line L3 (212.5056, 30) -> (208.7528, 36.5)
  line L4 (208.7528, 36.5) -> (201.2472, 36.5)
  line L5 (201.2472, 36.5) -> (197.4944, 30)
  constraints: 12 end point
extrude "Extrusion21" add sketch "Sketch_27" along normal blind 7
sketch "Sketch_28" plane through (0, 0, -80) normal (0, 0, 1) x (1, 0, 0)
  line L0 (-212.5056, 30) -> (-208.7528, 23.5)
  line L1 (-208.7528, 23.5) -> (-201.2472, 23.5)
  line L2 (-201.2472, 23.5) -> (-197.4944, 30)
  line L3 (-197.4944, 30) -> (-201.2472, 36.5)
  line L4 (-201.2472, 36.5) -> (-208.7528, 36.5)
  line L5 (-208.7528, 36.5) -> (-212.5056, 30)
  constraints: 12 end point
extrude "Extrusion22" add sketch "Sketch_28" along normal blind 7
sketch "Sketch_29" plane through (0, 0, -80) normal (0, 0, 1) x (1, 0, 0)
  line L0 (197.4944, 475) -> (201.2472, 468.5)
  line L1 (201.2472, 468.5) -> (208.7528, 468.5)
  line L2 (208.7528, 468.5) -> (212.5056, 475)
  line L3 (212.5056, 475) -> (208.7528, 481.5)
  line L4 (208.7528, 481.5) -> (201.2472, 481.5)
  line L5 (201.2472, 481.5) -> (197.4944, 475)
  constraints: 12 end point
extrude "Extrusion23" add sketch "Sketch_29" along normal blind 7
sketch "Sketch_30" plane through (0, 0, -80) normal (0, 0, 1) x (1, 0, 0)
  line L0 (-212.5056, 475) -> (-208.7528, 468.5)
  line L1 (-208.7528, 468.5) -> (-201.2472, 468.5)
  line L2 (-201.2472, 468.5) -> (-197.4944, 475)
  line L3 (-197.4944, 475) -> (-201.2472, 481.5)
  line L4 (-201.2472, 481.5) -> (-208.7528, 481.5)
  line L5 (-208.7528, 481.5) -> (-212.5056, 475)
  constraints: 12 end point
extrude "Extrusion24" add sketch "Sketch_30" along normal blind 7
ref_plane "DPB11_XY" through (250, 250, 0) normal (0, 0, 1) x (1, 0, 0)
ref_plane "DPB11_YZ" through (250, 250, 0) normal (1, 0, 0) x (0, 1, 0)
ref_plane "DPB11_ZX" through (250, 250, 0) normal (0, 1, 0) x (0, 0, 1)
ref_plane "DPB12_XY" through (-250, 250, 0) normal (0, 0, 1) x (1, 0, 0)
ref_plane "DPB12_YZ" through (-250, 250, 0) normal (1, 0, 0) x (0, 1, 0)
ref_plane "DPB12_ZX" through (-250, 250, 0) normal (0, 1, 0) x (0, 0, 1)
ref_plane "DPB61_XY" through (-151.5, 4, 0) normal (0, 0, 1) x (1, 0, 0)
ref_plane "DPB61_YZ" through (-151.5, 4, 0) normal (1, 0, 0) x (0, 1, 0)
ref_plane "DPB61_ZX" through (-151.5, 4, 0) normal (0, 1, 0) x (0, 0, 1)
ref_plane "DPB62_XY" through (151.5, 4, 0) normal (0, 0, 1) x (1, 0, 0)
ref_plane "DPB62_YZ" through (151.5, 4, 0) normal (1, 0, 0) x (0, 1, 0)
ref_plane "DPB62_ZX" through (151.5, 4, 0) normal (0, 1, 0) x (0, 0, 1)
ref_plane "DPH11_XY" through (0, 0, 0) normal (0, 0, 1) x (1, 0, 0)
ref_plane "DPH11_YZ" through (0, 0, 0) normal (1, 0, 0) x (0, 1, 0)
ref_plane "DPH11_ZX" through (0, 0, 0) normal (0, 1, 0) x (0, 0, 1)
ref_plane "DPH12_XY" through (0, 500, 0) normal (0, 0, 1) x (1, 0, 0)
ref_plane "DPH12_YZ" through (0, 500, 0) normal (1, 0, 0) x (0, 1, 0)
ref_plane "DPH12_ZX" through (0, 500, 0) normal (0, 1, 0) x (0, 0, 1)
ref_plane "DPH21_XY" through (0, 2.5, 105) normal (1, 0, 0) x (0, 0, -1)
ref_plane "DPH21_YZ" through (0, 2.5, 105) normal (0, 0, -1) x (0, 1, 0)
ref_plane "DPH21_ZX" through (0, 2.5, 105) normal (0, 1, 0) x (1, 0, 0)
ref_plane "DPH22_XY" through (0, 497.5, 105) normal (1, 0, 0) x (0, 0, -1)
ref_plane "DPH22_YZ" through (0, 497.5, 105) normal (0, 0, -1) x (0, 1, 0)
ref_plane "DPH22_ZX" through (0, 497.5, 105) normal (0, 1, 0) x (1, 0, 0)
ref_plane "DPH31_XY" through (0, 20, 91.8) normal (1, 0, 0) x (0, 0, -1)
ref_plane "DPH31_YZ" through (0, 20, 91.8) normal (0, 0, -1) x (0, 1, 0)
ref_plane "DPH31_ZX" through (0, 20, 91.8) normal (0, 1, 0) x (1, 0, 0)
ref_plane "DPH32_XY" through (0, 480, 91.8) normal (1, 0, 0) x (0, 0, -1)
ref_plane "DPH32_YZ" through (0, 480, 91.8) normal (0, 0, -1) x (0, 1, 0)
ref_plane "DPH32_ZX" through (0, 480, 91.8) normal (0, 1, 0) x (1, 0, 0)
ref_plane "DPH51_XY" through (0, 0, -105) normal (1, 0, 0) x (0, 0, -1)
ref_plane "DPH51_YZ" through (0, 0, -105) normal (0, 0, -1) x (0, 1, 0)
ref_plane "DPH51_ZX" through (0, 0, -105) normal (0, 1, 0) x (1, 0, 0)
ref_plane "DPH52_XY" through (0, 30, -105) normal (1, 0, 0) x (0, 0, -1)
ref_plane "DPH52_YZ" through (0, 30, -105) normal (0, 0, -1) x (0, 1, 0)
ref_plane "DPH52_ZX" through (0, 30, -105) normal (0, 1, 0) x (1, 0, 0)
ref_plane "DPH61_XY" through (0, 2.5, 105) normal (1, 0, 0) x (0, 0, -1)
ref_plane "DPH61_YZ" through (0, 2.5, 105) normal (0, 0, -1) x (0, 1, 0)
ref_plane "DPH61_ZX" through (0, 2.5, 105) normal (0, 1, 0) x (1, 0, 0)
ref_plane "DPH62_XY" through (0, 0, 85) normal (1, 0, 0) x (0, 0, -1)
ref_plane "DPH62_YZ" through (0, 0, 85) normal (0, 0, -1) x (0, 1, 0)
ref_plane "DPH62_ZX" through (0, 0, 85) normal (0, 1, 0) x (1, 0, 0)
ref_plane "DPT11_XY" through (0, 0, -105) normal (1, 0, 0) x (0, 0, -1)
ref_plane "DPT11_YZ" through (0, 0, -105) normal (0, 0, -1) x (0, 1, 0)
ref_plane "DPT11_ZX" through (0, 0, -105) normal (0, 1, 0) x (1, 0, 0)
ref_plane "DPT12_XY" through (0, 2.5, 105) normal (1, 0, 0) x (0, 0, -1)
ref_plane "DPT12_YZ" through (0, 2.5, 105) normal (0, 0, -1) x (0, 1, 0)
ref_plane "DPT12_ZX" through (0, 2.5, 105) normal (0, 1, 0) x (1, 0, 0)
ref_plane "DPT21_XY" through (0, 500, -105) normal (1, 0, 0) x (0, 0, -1)
ref_plane "DPT21_YZ" through (0, 500, -105) normal (0, 0, -1) x (0, 1, 0)
ref_plane "DPT21_ZX" through (0, 500, -105) normal (0, 1, 0) x (1, 0, 0)
ref_plane "DPT22_XY" through (0, 500, 85) normal (1, 0, 0) x (0, 0, -1)
ref_plane "DPT22_YZ" through (0, 500, 85) normal (0, 0, -1) x (0, 1, 0)
ref_plane "DPT22_ZX" through (0, 500, 85) normal (0, 1, 0) x (1, 0, 0)
ref_plane "DPT41_XY" through (0, 4, -105) normal (1, 0, 0) x (0, 0, -1)
ref_plane "DPT41_YZ" through (0, 4, -105) normal (0, 0, -1) x (0, 1, 0)
ref_plane "DPT41_ZX" through (0, 4, -105) normal (0, 1, 0) x (1, 0, 0)
ref_plane "DPT42_XY" through (0, 4, -67) normal (1, 0, 0) x (0, 0, -1)
ref_plane "DPT42_YZ" through (0, 4, -67) normal (0, 0, -1) x (0, 1, 0)
ref_plane "DPT42_ZX" through (0, 4, -67) normal (0, 1, 0) x (1, 0, 0)
ref_plane "DPT51_XY" through (0, 4, -67) normal (1, 0, 0) x (0, 0, -1)
ref_plane "DPT51_YZ" through (0, 4, -67) normal (0, 0, -1) x (0, 1, 0)
ref_plane "DPT51_ZX" through (0, 4, -67) normal (0, 1, 0) x (1, 0, 0)
ref_plane "DPT52_XY" through (0, 4, 46) normal (1, 0, 0) x (0, 0, -1)
ref_plane "DPT52_YZ" through (0, 4, 46) normal (0, 0, -1) x (0, 1, 0)
ref_plane "DPT52_ZX" through (0, 4, 46) normal (0, 1, 0) x (1, 0, 0)
ref_plane "flanschplatte_XY" through (0, 0, -10.5) normal (0, 1, 0) x (1, 0, 0)
ref_plane "flanschplatte_YZ" through (0, 0, -10.5) normal (1, 0, 0) x (0, 0, -1)
ref_plane "flanschplatte_ZX" through (0, 0, -10.5) normal (0, 0, -1) x (0, 1, 0)
ref_plane "flanschplatte_2_XY" through (0, 0, -10.5) normal (0, 1, 0) x (1, 0, 0)
ref_plane "flanschplatte_2_YZ" through (0, 0, -10.5) normal (1, 0, 0) x (0, 0, -1)
ref_plane "flanschplatte_2_ZX" through (0, 0, -10.5) normal (0, 0, -1) x (0, 1, 0)
ref_plane "gehaeuse_XY" through (0, 0, 0) normal (0, 1, 0) x (1, 0, 0)
ref_plane "gehaeuse_YZ" through (0, 0, 0) normal (1, 0, 0) x (0, 0, -1)
ref_plane "gehaeuse_ZX" through (0, 0, 0) normal (0, 0, -1) x (0, 1, 0)
ref_plane "montageplatte_XY" through (-205, 30, -81) normal (0, 0, 1) x (1, 0, 0)
ref_plane "montageplatte_YZ" through (-205, 30, -81) normal (1, 0, 0) x (0, 1, 0)
ref_plane "montageplatte_ZX" through (-205, 30, -81) normal (0, 1, 0) x (0, 0, 1)
ref_plane "scharnier_o_XY" through (240.3, 431.85, 85) normal (0, 0, 1) x (1, 0, 0)
ref_plane "scharnier_o_YZ" through (240.3, 431.85, 85) normal (1, 0, 0) x (0, 1, 0)
ref_plane "scharnier_o_ZX" through (240.3, 431.85, 85) normal (0, 1, 0) x (0, 0, 1)
ref_plane "scharnier_u_XY" through (240.3, 50.65, 85) normal (0, 0, 1) x (1, 0, 0)
ref_plane "scharnier_u_YZ" through (240.3, 50.65, 85) normal (1, 0, 0) x (0, 1, 0)
ref_plane "scharnier_u_ZX" through (240.3, 50.65, 85) normal (0, 1, 0) x (0, 0, 1)
body "Solid1"
